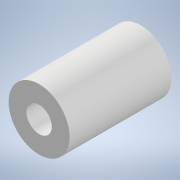
# Autodesk Inventor part: motorCoupling5_8
Saved by Autodesk Inventor 2020 (Build 240168000, 168)
## iProperties
Created: 2022-12-14
Part Number: motorCoupling5_8
Material: Generic
Document SubType Name: Modeling
Designer: Manish
Density: 1 g/cm^3
Appearance: Default
Author: Manish
Autodesk Inventor part; units mm, degrees
ref_plane "YZ Plane" through (0, 0, 0) normal (1, 0, 0) x (0, 1, 0)
ref_plane "XZ Plane" through (0, 0, 0) normal (0, 1, 0) x (-1, 0, 0)
ref_plane "XY Plane" through (0, 0, 0) normal (0, 0, 1) x (1, 0, 0)
sketch "Sketch1" plane through (0, 0, 0) normal (0, 1, 0) x (-1, 0, 0)
  line L0 (0, 0) -> (-6, 0)
  line L1 (-6, 0) -> (-6, -20)
  line L2 (-6, -20) -> (0, -20)
  line L3 (0, -20) -> (0, 0)
  line L4 (0, 0) -> (-2.5, 0)
  line L5 (0, -10) -> (-2.5, -10)
  line L6 (-2.5, -8) -> (-2.5, 0)
  line L7 (0, -20) -> (-4, -20)
  line L8 (-4, -20) -> (-4, -11.1225)
  line L9 (-4, -10) -> (-4.5, -10)
  arc A0 (-3.25, -9.5612) -> (-2.5, -8) centre (-4.5, -8) ccw
  arc A1 (-3.25, -9.5612) -> (-4, -11.1225) centre (-2, -11.1225) ccw
  dimension "d0" = 6
  dimension "d1" = 20
  dimension "d2" = 2.5
  dimension "d3" = 4
  dimension "d4" = 2
  constraints: 20 end point, 6 point on line, 5 perpendicular, 5 point on circle, 4 tangent, 2 centre point, 2 horizontal, 1 equal radius, 1 midpoint, 1 vertical
  measures "d0" distance of L0.start L0.end
  measures "d1" distance of L0.end L1.end
  measures "d2" distance of L0.start L4.end
  measures "d3" distance of L2.end L7.end
  measures "d4" radius of A0
revolve "Revolution1" add sketch "Sketch1" angle 360 about axis through (0, 0, -20) along (0, 0, 1) contours L6 A0 A1 L8 L2 L1 L0
ref_plane "Work Plane1" through (0, 0, -10) normal (0, 0, 1) x (1, 0, 0)
body "Solid1"
